Autodesk Fusion 360 part; units mm, degrees
(part 26 of 40)
  line L4946 (24.3039, -56.3229) -> (24.3478, -56.4711) construction
  line L4947 (24.3478, -56.4711) -> (24.3873, -56.6208) construction
  line L4948 (24.3873, -56.6208) -> (24.4241, -56.7714) construction
  line L4949 (24.4241, -56.7714) -> (24.4595, -56.9226) construction
  line L4950 (24.4595, -56.9226) -> (24.494, -57.0741) construction
  line L4951 (24.494, -57.0741) -> (24.5274, -57.226) construction
  line L4952 (24.5274, -57.226) -> (24.5594, -57.3783) construction
  line L4953 (24.5594, -57.3783) -> (24.5896, -57.5312) construction
  line L4954 (24.5896, -57.5312) -> (24.6176, -57.6848) construction
  line L4955 (24.6176, -57.6848) -> (24.6435, -57.8391) construction
  line L4956 (24.6435, -57.8391) -> (24.6674, -57.994) construction
  line L4957 (24.6674, -57.994) -> (24.6897, -58.1494) construction
  line L4958 (24.6897, -58.1494) -> (24.7105, -58.3052) construction
  line L4959 (24.7105, -58.3052) -> (24.7301, -58.4614) construction
  line L4960 (24.7301, -58.4614) -> (24.7485, -58.6179) construction
  line L4961 (24.7485, -58.6179) -> (24.7658, -58.7747) construction
  line L4962 (24.7658, -58.7747) -> (24.7818, -58.9318) construction
  line L4963 (24.7818, -58.9318) -> (24.7965, -59.0893) construction
  line L4964 (24.7965, -59.0893) -> (24.8098, -59.2471) construction
  line L4965 (24.8098, -59.2471) -> (24.8218, -59.4053) construction
  line L4966 (24.8218, -59.4053) -> (24.8325, -59.5638) construction
  line L4967 (24.8325, -59.5638) -> (24.842, -59.7226) construction
  line L4968 (24.842, -59.7226) -> (24.8504, -59.8817) construction
  line L4969 (24.8504, -59.8817) -> (24.8577, -60.0411) construction
  line L4970 (24.8577, -60.0411) -> (24.8638, -60.2007) construction
  line L4971 (24.8638, -60.2007) -> (24.8689, -60.3605) construction
  line L4972 (24.8689, -60.3605) -> (24.8729, -60.5206) construction
  line L4973 (24.8729, -60.5206) -> (24.8757, -60.6809) construction
  line L4974 (24.8757, -60.6809) -> (24.8776, -60.8415) construction
  line L4975 (24.8776, -60.8415) -> (24.8783, -61.0023) construction
  line L4976 (24.8783, -61.0023) -> (24.878, -61.1633) construction
  line L4977 (24.878, -61.1633) -> (24.8766, -61.3245) construction
  line L4978 (24.8766, -61.3245) -> (24.8742, -61.4859) construction
  line L4979 (24.8742, -61.4859) -> (24.8708, -61.6475) construction
  line L4980 (24.8708, -61.6475) -> (24.8665, -61.8093) construction
  line L4981 (24.8665, -61.8093) -> (24.8611, -61.9712) construction
  line L4982 (24.8611, -61.9712) -> (24.8548, -62.1334) construction
  line L4983 (24.8548, -62.1334) -> (24.8475, -62.2957) construction
  line L4984 (24.8475, -62.2957) -> (24.8392, -62.4581) construction
  line L4985 (24.8392, -62.4581) -> (24.83, -62.6207) construction
  line L4986 (24.83, -62.6207) -> (24.8199, -62.7835) construction
  line L4987 (24.8199, -62.7835) -> (24.8088, -62.9464) construction
  line L4988 (24.8088, -62.9464) -> (24.7967, -63.1095) construction
  line L4989 (24.7967, -63.1095) -> (24.7838, -63.2727) construction
  line L4990 (24.7838, -63.2727) -> (24.77, -63.436) construction
  line L4991 (24.77, -63.436) -> (24.7552, -63.5995) construction
  line L4992 (24.7552, -63.5995) -> (24.7396, -63.7631) construction
  line L4993 (24.7396, -63.7631) -> (24.723, -63.9268) construction
  line L4994 (24.723, -63.9268) -> (24.7056, -64.0906) construction
  line L4995 (24.7056, -64.0906) -> (24.6873, -64.2545) construction
  line L4996 (24.6873, -64.2545) -> (24.6681, -64.4185) construction
  line L4997 (24.6681, -64.4185) -> (24.648, -64.5826) construction
  line L4998 (24.648, -64.5826) -> (24.6271, -64.7468) construction
  line L4999 (24.6271, -64.7468) -> (24.6054, -64.9111) construction
  line L5000 (24.6054, -64.9111) -> (24.5828, -65.0755) construction
  line L5001 (24.5828, -65.0755) -> (24.5593, -65.24) construction
  line L5002 (24.5593, -65.24) -> (24.535, -65.4046) construction
  line L5003 (24.535, -65.4046) -> (24.5098, -65.5692) construction
  line L5004 (24.5098, -65.5692) -> (24.4839, -65.734) construction
  line L5005 (24.4839, -65.734) -> (24.4571, -65.8987) construction
  line L5006 (24.4571, -65.8987) -> (24.4294, -66.0636) construction
  line L5007 (24.4294, -66.0636) -> (24.401, -66.2285) construction
  line L5008 (24.401, -66.2285) -> (24.3718, -66.3935) construction
  line L5009 (24.3718, -66.3935) -> (24.3417, -66.5585) construction
  line L5010 (24.3417, -66.5585) -> (24.3108, -66.7236) construction
  line L5011 (24.3108, -66.7236) -> (24.2792, -66.8887) construction
  line L5012 (24.2792, -66.8887) -> (24.2532, -67.0208) construction
  line L5013 (24.2532, -67.0208) -> (24.2334, -67.1199) construction
  line L5014 (24.2334, -67.1199) -> (24.22, -67.186) construction
  line L5015 (24.22, -67.186) -> (24.2132, -67.2191) construction
  line L5016 (-59.1442, 5.5428) -> (-60.7685, 5.6951)
  line L5017 (-30.2798, 51.1066) -> (-31.1115, 52.5103)
  line L5018 (57.9623, -13.005) -> (59.5542, -13.3622)
  line L5019 (-13.005, 57.9623) -> (-13.3622, 59.5542)
  arc A123 (-54.5366, 23.5481) -> (-51.9354, 24.5301) centre (-53.7438, 25.3842) ccw
  arc A124 (56.9737, 7.2806) -> (59.1442, 5.5428) centre (58.9575, 7.5341) ccw
  arc A125 (-39.3784, 41.8132) -> (-39.2483, 44.5906) centre (-40.7496, 43.2692) ccw
  spline S67 degree 5 poles (-40.3263, 45.8153) (-40.3467, 45.8385) (-40.3868, 45.8854) (-40.4451, 45.9573) (-40.5192, 46.056) (-40.6066, 46.1833) (-40.6904, 46.3135) (-40.772, 46.4454) (-40.8524, 46.5782) (-40.932, 46.7117) (-41.0107, 46.8458) (-41.0883, 46.9807) (-41.1642, 47.1168) (-41.2383, 47.2543) (-41.3106, 47.393) (-41.3813, 47.5329) (-41.4504, 47.6738) (-41.5184, 47.8156) (-41.5853, 47.9581) (-41.6512, 48.1012) (-41.716, 48.245) (-41.7798, 48.3895) (-41.8424, 48.5347) (-41.9039, 48.6807) (-41.9642, 48.8274) (-42.0234, 48.9749) (-42.0815, 49.123) (-42.1386, 49.2717) (-42.1947, 49.421) (-42.2499, 49.5709) (-42.3041, 49.7214) (-42.3574, 49.8724) (-42.4097, 50.024) (-42.461, 50.1761) (-42.5114, 50.3288) (-42.5608, 50.482) (-42.6094, 50.6358) (-42.657, 50.79) (-42.7037, 50.9447) (-42.7495, 51.0999) (-42.7945, 51.2556) (-42.8386, 51.4118) (-42.8818, 51.5684) (-42.9241, 51.7255) (-42.9656, 51.883) (-43.0063, 52.0409) (-43.0461, 52.1993) (-43.085, 52.3581) (-43.1231, 52.5173) (-43.1604, 52.6769) (-43.1969, 52.8369) (-43.2326, 52.9973) (-43.2674, 53.1581) (-43.3015, 53.3193) (-43.3347, 53.4809) (-43.3672, 53.6428) (-43.3988, 53.8051) (-43.4297, 53.9677) (-43.4597, 54.1307) (-43.489, 54.294) (-43.5175, 54.4577) (-43.5453, 54.6217) (-43.5723, 54.7861) (-43.5984, 54.9508) (-43.6239, 55.1158) (-43.6486, 55.2811) (-43.6725, 55.4467) (-43.6956, 55.6126) (-43.718, 55.7789) (-43.7397, 55.9454) (-43.7606, 56.1122) (-43.7767, 56.2459) (-43.7885, 56.3463) (-43.7962, 56.4133) (-43.8, 56.4469) knots 0 0 0 0 0 0 0.01428571 0.02857143 0.04285714 0.05714286 0.07142857 0.08571429 0.1 0.11428571 0.12857143 0.14285714 0.15714286 0.17142857 0.18571429 0.2 0.21428571 0.22857143 0.24285714 0.25714286 0.27142857 0.28571429 0.3 0.31428571 0.32857143 0.34285714 0.35714286 0.37142857 0.38571429 0.4 0.41428571 0.42857143 0.44285714 0.45714286 0.47142857 0.48571429 0.5 0.51428571 0.52857143 0.54285714 0.55714286 0.57142857 0.58571429 0.6 0.61428571 0.62857143 0.64285714 0.65714286 0.67142857 0.68571429 0.7 0.71428571 0.72857143 0.74285714 0.75714286 0.77142857 0.78571429 0.8 0.81428571 0.82857143 0.84285714 0.85714286 0.87142857 0.88571429 0.9 0.91428571 0.92857143 0.94285714 0.95714286 0.97142857 0.98571429 1 1 1 1 1 1
  line L5020 (-40.3263, 45.8153) -> (-40.3467, 45.8385) construction
  line L5021 (-40.3467, 45.8385) -> (-40.3868, 45.8854) construction
  line L5022 (-40.3868, 45.8854) -> (-40.4451, 45.9573) construction
  line L5023 (-40.4451, 45.9573) -> (-40.5192, 46.056) construction
  line L5024 (-40.5192, 46.056) -> (-40.6066, 46.1833) construction
  line L5025 (-40.6066, 46.1833) -> (-40.6904, 46.3135) construction
  line L5026 (-40.6904, 46.3135) -> (-40.772, 46.4454) construction
  line L5027 (-40.772, 46.4454) -> (-40.8524, 46.5782) construction
  line L5028 (-40.8524, 46.5782) -> (-40.932, 46.7117) construction
  line L5029 (-40.932, 46.7117) -> (-41.0107, 46.8458) construction
  line L5030 (-41.0107, 46.8458) -> (-41.0883, 46.9807) construction
  line L5031 (-41.0883, 46.9807) -> (-41.1642, 47.1168) construction
  line L5032 (-41.1642, 47.1168) -> (-41.2383, 47.2543) construction
  line L5033 (-41.2383, 47.2543) -> (-41.3106, 47.393) construction
  line L5034 (-41.3106, 47.393) -> (-41.3813, 47.5329) construction
  line L5035 (-41.3813, 47.5329) -> (-41.4504, 47.6738) construction
  line L5036 (-41.4504, 47.6738) -> (-41.5184, 47.8156) construction
  line L5037 (-41.5184, 47.8156) -> (-41.5853, 47.9581) construction
  line L5038 (-41.5853, 47.9581) -> (-41.6512, 48.1012) construction
  line L5039 (-41.6512, 48.1012) -> (-41.716, 48.245) construction
  line L5040 (-41.716, 48.245) -> (-41.7798, 48.3895) construction
  line L5041 (-41.7798, 48.3895) -> (-41.8424, 48.5347) construction
  line L5042 (-41.8424, 48.5347) -> (-41.9039, 48.6807) construction
  line L5043 (-41.9039, 48.6807) -> (-41.9642, 48.8274) construction
  line L5044 (-41.9642, 48.8274) -> (-42.0234, 48.9749) construction
  line L5045 (-42.0234, 48.9749) -> (-42.0815, 49.123) construction
  line L5046 (-42.0815, 49.123) -> (-42.1386, 49.2717) construction
  line L5047 (-42.1386, 49.2717) -> (-42.1947, 49.421) construction
  line L5048 (-42.1947, 49.421) -> (-42.2499, 49.5709) construction
  line L5049 (-42.2499, 49.5709) -> (-42.3041, 49.7214) construction
  line L5050 (-42.3041, 49.7214) -> (-42.3574, 49.8724) construction
  line L5051 (-42.3574, 49.8724) -> (-42.4097, 50.024) construction
  line L5052 (-42.4097, 50.024) -> (-42.461, 50.1761) construction
  line L5053 (-42.461, 50.1761) -> (-42.5114, 50.3288) construction
  line L5054 (-42.5114, 50.3288) -> (-42.5608, 50.482) construction
  line L5055 (-42.5608, 50.482) -> (-42.6094, 50.6358) construction
  line L5056 (-42.6094, 50.6358) -> (-42.657, 50.79) construction
  line L5057 (-42.657, 50.79) -> (-42.7037, 50.9447) construction
  line L5058 (-42.7037, 50.9447) -> (-42.7495, 51.0999) construction
  line L5059 (-42.7495, 51.0999) -> (-42.7945, 51.2556) construction
  line L5060 (-42.7945, 51.2556) -> (-42.8386, 51.4118) construction
  line L5061 (-42.8386, 51.4118) -> (-42.8818, 51.5684) construction
  line L5062 (-42.8818, 51.5684) -> (-42.9241, 51.7255) construction
  line L5063 (-42.9241, 51.7255) -> (-42.9656, 51.883) construction
  line L5064 (-42.9656, 51.883) -> (-43.0063, 52.0409) construction
  line L5065 (-43.0063, 52.0409) -> (-43.0461, 52.1993) construction
  line L5066 (-43.0461, 52.1993) -> (-43.085, 52.3581) construction
  line L5067 (-43.085, 52.3581) -> (-43.1231, 52.5173) construction
  line L5068 (-43.1231, 52.5173) -> (-43.1604, 52.6769) construction
  line L5069 (-43.1604, 52.6769) -> (-43.1969, 52.8369) construction
  line L5070 (-43.1969, 52.8369) -> (-43.2326, 52.9973) construction
  line L5071 (-43.2326, 52.9973) -> (-43.2674, 53.1581) construction
  line L5072 (-43.2674, 53.1581) -> (-43.3015, 53.3193) construction
  line L5073 (-43.3015, 53.3193) -> (-43.3347, 53.4809) construction
  line L5074 (-43.3347, 53.4809) -> (-43.3672, 53.6428) construction
  line L5075 (-43.3672, 53.6428) -> (-43.3988, 53.8051) construction
  line L5076 (-43.3988, 53.8051) -> (-43.4297, 53.9677) construction
  line L5077 (-43.4297, 53.9677) -> (-43.4597, 54.1307) construction
  line L5078 (-43.4597, 54.1307) -> (-43.489, 54.294) construction
  line L5079 (-43.489, 54.294) -> (-43.5175, 54.4577) construction
  line L5080 (-43.5175, 54.4577) -> (-43.5453, 54.6217) construction
  line L5081 (-43.5453, 54.6217) -> (-43.5723, 54.7861) construction
  line L5082 (-43.5723, 54.7861) -> (-43.5984, 54.9508) construction
  line L5083 (-43.5984, 54.9508) -> (-43.6239, 55.1158) construction
  line L5084 (-43.6239, 55.1158) -> (-43.6486, 55.2811) construction
  line L5085 (-43.6486, 55.2811) -> (-43.6725, 55.4467) construction
  line L5086 (-43.6725, 55.4467) -> (-43.6956, 55.6126) construction
  line L5087 (-43.6956, 55.6126) -> (-43.718, 55.7789) construction
  line L5088 (-43.718, 55.7789) -> (-43.7397, 55.9454) construction
  line L5089 (-43.7397, 55.9454) -> (-43.7606, 56.1122) construction
  line L5090 (-43.7606, 56.1122) -> (-43.7767, 56.2459) construction
  line L5091 (-43.7767, 56.2459) -> (-43.7885, 56.3463) construction
  line L5092 (-43.7885, 56.3463) -> (-43.7962, 56.4133) construction
  line L5093 (-43.7962, 56.4133) -> (-43.8, 56.4469) construction
  arc A126 (24.2132, 67.2191) -> (19.9215, 68.6136) centre (0, 0) ccw
  spline S68 degree 5 poles (5.6951, 60.7685) (5.6979, 60.7993) (5.7029, 60.8609) (5.7078, 60.9533) (5.7097, 61.0766) (5.7056, 61.231) (5.6969, 61.3856) (5.6854, 61.5403) (5.6723, 61.695) (5.6583, 61.8498) (5.6431, 62.0045) (5.6265, 62.1593) (5.608, 62.314) (5.5871, 62.4688) (5.5641, 62.6235) (5.539, 62.7782) (5.5121, 62.9329) (5.4838, 63.0875) (5.4542, 63.2421) (5.4233, 63.3966) (5.3913, 63.5511) (5.3579, 63.7055) (5.3232, 63.8598) (5.2871, 64.014) (5.2497, 64.1682) (5.2109, 64.3222) (5.1709, 64.4762) (5.1297, 64.6301) (5.0873, 64.7839) (5.0439, 64.9376) (4.9993, 65.0912) (4.9536, 65.2447) (4.9068, 65.398) (4.8589, 65.5513) (4.8099, 65.7044) (4.7599, 65.8574) (4.7087, 66.0103) (4.6566, 66.1631) (4.6035, 66.3158) (4.5493, 66.4683) (4.4942, 66.6206) (4.438, 66.7729) (4.381, 66.925) (4.3229, 67.077) (4.2639, 67.2288) (4.2039, 67.3804) (4.143, 67.532) (4.0812, 67.6833) (4.0185, 67.8345) (3.9548, 67.9856) (3.8903, 68.1365) (3.8249, 68.2872) (3.7585, 68.4378) (3.6913, 68.5882) (3.6233, 68.7384) (3.5543, 68.8885) (3.4846, 69.0384) (3.4139, 69.1881) (3.3425, 69.3376) (3.2701, 69.487) (3.197, 69.6362) (3.123, 69.7852) (3.0482, 69.934) (2.9726, 70.0826) (2.8962, 70.2311) (2.819, 70.3793) (2.741, 70.5274) (2.6622, 70.6752) (2.5826, 70.8229) (2.5023, 70.9703) (2.4211, 71.1176) (2.3556, 71.2352) (2.3061, 71.3234) (2.2729, 71.3821) (2.2563, 71.4115) knots 0 0 0 0 0 0 0.01428571 0.02857143 0.04285714 0.05714286 0.07142857 0.08571429 0.1 0.11428571 0.12857143 0.14285714 0.15714286 0.17142857 0.18571429 0.2 0.21428571 0.22857143 0.24285714 0.25714286 0.27142857 0.28571429 0.3 0.31428571 0.32857143 0.34285714 0.35714286 0.37142857 0.38571429 0.4 0.41428571 0.42857143 0.44285714 0.45714286 0.47142857 0.48571429 0.5 0.51428571 0.52857143 0.54285714 0.55714286 0.57142857 0.58571429 0.6 0.61428571 0.62857143 0.64285714 0.65714286 0.67142857 0.68571429 0.7 0.71428571 0.72857143 0.74285714 0.75714286 0.77142857 0.78571429 0.8 0.81428571 0.82857143 0.84285714 0.85714286 0.87142857 0.88571429 0.9 0.91428571 0.92857143 0.94285714 0.95714286 0.97142857 0.98571429 1 1 1 1 1 1
  line L5094 (5.6951, 60.7685) -> (5.6979, 60.7993) construction
  line L5095 (5.6979, 60.7993) -> (5.7029, 60.8609) construction
  line L5096 (5.7029, 60.8609) -> (5.7078, 60.9533) construction
  line L5097 (5.7078, 60.9533) -> (5.7097, 61.0766) construction
  line L5098 (5.7097, 61.0766) -> (5.7056, 61.231) construction
  line L5099 (5.7056, 61.231) -> (5.6969, 61.3856) construction
  line L5100 (5.6969, 61.3856) -> (5.6854, 61.5403) construction
  line L5101 (5.6854, 61.5403) -> (5.6723, 61.695) construction
  line L5102 (5.6723, 61.695) -> (5.6583, 61.8498) construction
  line L5103 (5.6583, 61.8498) -> (5.6431, 62.0045) construction
  line L5104 (5.6431, 62.0045) -> (5.6265, 62.1593) construction
  line L5105 (5.6265, 62.1593) -> (5.608, 62.314) construction
  line L5106 (5.608, 62.314) -> (5.5871, 62.4688) construction
  line L5107 (5.5871, 62.4688) -> (5.5641, 62.6235) construction
  line L5108 (5.5641, 62.6235) -> (5.539, 62.7782) construction
  line L5109 (5.539, 62.7782) -> (5.5121, 62.9329) construction
  line L5110 (5.5121, 62.9329) -> (5.4838, 63.0875) construction
  line L5111 (5.4838, 63.0875) -> (5.4542, 63.2421) construction
  line L5112 (5.4542, 63.2421) -> (5.4233, 63.3966) construction
  line L5113 (5.4233, 63.3966) -> (5.3913, 63.5511) construction
  line L5114 (5.3913, 63.5511) -> (5.3579, 63.7055) construction
  line L5115 (5.3579, 63.7055) -> (5.3232, 63.8598) construction
  line L5116 (5.3232, 63.8598) -> (5.2871, 64.014) construction
  line L5117 (5.2871, 64.014) -> (5.2497, 64.1682) construction
  line L5118 (5.2497, 64.1682) -> (5.2109, 64.3222) construction
  line L5119 (5.2109, 64.3222) -> (5.1709, 64.4762) construction
  line L5120 (5.1709, 64.4762) -> (5.1297, 64.6301) construction
  line L5121 (5.1297, 64.6301) -> (5.0873, 64.7839) construction
  line L5122 (5.0873, 64.7839) -> (5.0439, 64.9376) construction
  line L5123 (5.0439, 64.9376) -> (4.9993, 65.0912) construction
  line L5124 (4.9993, 65.0912) -> (4.9536, 65.2447) construction
  line L5125 (4.9536, 65.2447) -> (4.9068, 65.398) construction
  line L5126 (4.9068, 65.398) -> (4.8589, 65.5513) construction
  line L5127 (4.8589, 65.5513) -> (4.8099, 65.7044) construction
  line L5128 (4.8099, 65.7044) -> (4.7599, 65.8574) construction
  line L5129 (4.7599, 65.8574) -> (4.7087, 66.0103) construction
  line L5130 (4.7087, 66.0103) -> (4.6566, 66.1631) construction
  line L5131 (4.6566, 66.1631) -> (4.6035, 66.3158) construction
  line L5132 (4.6035, 66.3158) -> (4.5493, 66.4683) construction
  line L5133 (4.5493, 66.4683) -> (4.4942, 66.6206) construction
  line L5134 (4.4942, 66.6206) -> (4.438, 66.7729) construction
  line L5135 (4.438, 66.7729) -> (4.381, 66.925) construction
  line L5136 (4.381, 66.925) -> (4.3229, 67.077) construction
  line L5137 (4.3229, 67.077) -> (4.2639, 67.2288) construction
  line L5138 (4.2639, 67.2288) -> (4.2039, 67.3804) construction
  line L5139 (4.2039, 67.3804) -> (4.143, 67.532) construction
  line L5140 (4.143, 67.532) -> (4.0812, 67.6833) construction
  line L5141 (4.0812, 67.6833) -> (4.0185, 67.8345) construction
  line L5142 (4.0185, 67.8345) -> (3.9548, 67.9856) construction
  line L5143 (3.9548, 67.9856) -> (3.8903, 68.1365) construction
  line L5144 (3.8903, 68.1365) -> (3.8249, 68.2872) construction
  line L5145 (3.8249, 68.2872) -> (3.7585, 68.4378) construction
  line L5146 (3.7585, 68.4378) -> (3.6913, 68.5882) construction
  line L5147 (3.6913, 68.5882) -> (3.6233, 68.7384) construction
  line L5148 (3.6233, 68.7384) -> (3.5543, 68.8885) construction
  line L5149 (3.5543, 68.8885) -> (3.4846, 69.0384) construction
  line L5150 (3.4846, 69.0384) -> (3.4139, 69.1881) construction
  line L5151 (3.4139, 69.1881) -> (3.3425, 69.3376) construction
  line L5152 (3.3425, 69.3376) -> (3.2701, 69.487) construction
  line L5153 (3.2701, 69.487) -> (3.197, 69.6362) construction
  line L5154 (3.197, 69.6362) -> (3.123, 69.7852) construction
  line L5155 (3.123, 69.7852) -> (3.0482, 69.934) construction
  line L5156 (3.0482, 69.934) -> (2.9726, 70.0826) construction
  line L5157 (2.9726, 70.0826) -> (2.8962, 70.2311) construction
  line L5158 (2.8962, 70.2311) -> (2.819, 70.3793) construction
  line L5159 (2.819, 70.3793) -> (2.741, 70.5274) construction
  line L5160 (2.741, 70.5274) -> (2.6622, 70.6752) construction
  line L5161 (2.6622, 70.6752) -> (2.5826, 70.8229) construction
  line L5162 (2.5826, 70.8229) -> (2.5023, 70.9703) construction
  line L5163 (2.5023, 70.9703) -> (2.4211, 71.1176) construction
  line L5164 (2.4211, 71.1176) -> (2.3556, 71.2352) construction
  line L5165 (2.3556, 71.2352) -> (2.3061, 71.3234) construction
  line L5166 (2.3061, 71.3234) -> (2.2729, 71.3821) construction
  line L5167 (2.2729, 71.3821) -> (2.2563, 71.4115) construction
  arc A127 (-41.8132, -39.3784) -> (-44.5906, -39.2483) centre (-43.2692, -40.7496) ccw
  arc A128 (39.3784, -41.8132) -> (39.2483, -44.5906) centre (40.7496, -43.2692) ccw
  arc A129 (54.5366, -23.5481) -> (51.9354, -24.5301) centre (53.7438, -25.3842) ccw
  spline S69 degree 5 poles (-31.1115, 52.5103) (-31.1272, 52.5368) (-31.1594, 52.5895) (-31.2097, 52.6672) (-31.2807, 52.7681) (-31.3748, 52.8906) (-31.4727, 53.0106) (-31.5729, 53.1289) (-31.6744, 53.2464) (-31.7767, 53.3634) (-31.88, 53.4797) (-31.9844, 53.5951) (-32.0903, 53.7094) (-32.1981, 53.8224) (-32.3077, 53.934) (-32.419, 54.0444) (-32.5316, 54.1537) (-32.6455, 54.2622) (-32.7603, 54.3698) (-32.876, 54.4767) (-32.9927, 54.5828) (-33.1105, 54.6881) (-33.2292, 54.7926) (-33.3491, 54.8961) (-33.47, 54.9988) (-33.5919, 55.1007) (-33.7148, 55.2017) (-33.8386, 55.302) (-33.9633, 55.4015) (-34.0888, 55.5003) (-34.2151, 55.5984) (-34.3423, 55.6957) (-34.4703, 55.7923) (-34.5991, 55.8881) (-34.7288, 55.9832) (-34.8592, 56.0776) (-34.9905, 56.1712) (-35.1224, 56.2642) (-35.2552, 56.3564) (-35.3886, 56.448) (-35.5228, 56.5388) (-35.6577, 56.629) (-35.7933, 56.7185) (-35.9295, 56.8073) (-36.0665, 56.8955) (-36.2042, 56.9829) (-36.3425, 57.0697) (-36.4815, 57.1558) (-36.6211, 57.2413) (-36.7614, 57.3261) (-36.9023, 57.4102) (-37.0438, 57.4937) (-37.186, 57.5765) (-37.3288, 57.6587) (-37.4721, 57.7403) (-37.6161, 57.8212) (-37.7607, 57.9014) (-37.9058, 57.981) (-38.0515, 58.06) (-38.1978, 58.1383) (-38.3447, 58.216) (-38.4921, 58.2931) (-38.6401, 58.3695) (-38.7886, 58.4453) (-38.9377, 58.5205) (-39.0873, 58.595) (-39.2374, 58.669) (-39.3881, 58.7423) (-39.5393, 58.8149) (-39.6909, 58.887) (-39.8431, 58.9584) (-39.9653, 59.0151) (-40.0572, 59.0573) (-40.1185, 59.0853) (-40.1492, 59.0993) knots 0 0 0 0 0 0 0.01428571 0.02857143 0.04285714 0.05714286 0.07142857 0.08571429 0.1 0.11428571 0.12857143 0.14285714 0.15714286 0.17142857 0.18571429 0.2 0.21428571 0.22857143 0.24285714 0.25714286 0.27142857 0.28571429 0.3 0.31428571 0.32857143 0.34285714 0.35714286 0.37142857 0.38571429 0.4 0.41428571 0.42857143 0.44285714 0.45714286 0.47142857 0.48571429 0.5 0.51428571 0.52857143 0.54285714 0.55714286 0.57142857 0.58571429 0.6 0.61428571 0.62857143 0.64285714 0.65714286 0.67142857 0.68571429 0.7 0.71428571 0.72857143 0.74285714 0.75714286 0.77142857 0.78571429 0.8 0.81428571 0.82857143 0.84285714 0.85714286 0.87142857 0.88571429 0.9 0.91428571 0.92857143 0.94285714 0.95714286 0.97142857 0.98571429 1 1 1 1 1 1
  line L5168 (-31.1115, 52.5103) -> (-31.1272, 52.5368) construction
  line L5169 (-31.1272, 52.5368) -> (-31.1594, 52.5895) construction
  line L5170 (-31.1594, 52.5895) -> (-31.2097, 52.6672) construction
  line L5171 (-31.2097, 52.6672) -> (-31.2807, 52.7681) construction
  line L5172 (-31.2807, 52.7681) -> (-31.3748, 52.8906) construction
  line L5173 (-31.3748, 52.8906) -> (-31.4727, 53.0106) construction
  line L5174 (-31.4727, 53.0106) -> (-31.5729, 53.1289) construction
  line L5175 (-31.5729, 53.1289) -> (-31.6744, 53.2464) construction
  line L5176 (-31.6744, 53.2464) -> (-31.7767, 53.3634) construction
  line L5177 (-31.7767, 53.3634) -> (-31.88, 53.4797) construction
  line L5178 (-31.88, 53.4797) -> (-31.9844, 53.5951) construction
  line L5179 (-31.9844, 53.5951) -> (-32.0903, 53.7094) construction
  line L5180 (-32.0903, 53.7094) -> (-32.1981, 53.8224) construction
  line L5181 (-32.1981, 53.8224) -> (-32.3077, 53.934) construction
  line L5182 (-32.3077, 53.934) -> (-32.419, 54.0444) construction
  line L5183 (-32.419, 54.0444) -> (-32.5316, 54.1537) construction
  line L5184 (-32.5316, 54.1537) -> (-32.6455, 54.2622) construction
  line L5185 (-32.6455, 54.2622) -> (-32.7603, 54.3698) construction
  line L5186 (-32.7603, 54.3698) -> (-32.876, 54.4767) construction
  line L5187 (-32.876, 54.4767) -> (-32.9927, 54.5828) construction
  line L5188 (-32.9927, 54.5828) -> (-33.1105, 54.6881) construction
  line L5189 (-33.1105, 54.6881) -> (-33.2292, 54.7926) construction
  line L5190 (-33.2292, 54.7926) -> (-33.3491, 54.8961) construction
  line L5191 (-33.3491, 54.8961) -> (-33.47, 54.9988) construction
  line L5192 (-33.47, 54.9988) -> (-33.5919, 55.1007) construction
  line L5193 (-33.5919, 55.1007) -> (-33.7148, 55.2017) construction
  line L5194 (-33.7148, 55.2017) -> (-33.8386, 55.302) construction
  line L5195 (-33.8386, 55.302) -> (-33.9633, 55.4015) construction
  line L5196 (-33.9633, 55.4015) -> (-34.0888, 55.5003) construction
  line L5197 (-34.0888, 55.5003) -> (-34.2151, 55.5984) construction
  line L5198 (-34.2151, 55.5984) -> (-34.3423, 55.6957) construction
  line L5199 (-34.3423, 55.6957) -> (-34.4703, 55.7923) construction
  line L5200 (-34.4703, 55.7923) -> (-34.5991, 55.8881) construction
  line L5201 (-34.5991, 55.8881) -> (-34.7288, 55.9832) construction
  line L5202 (-34.7288, 55.9832) -> (-34.8592, 56.0776) construction
  line L5203 (-34.8592, 56.0776) -> (-34.9905, 56.1712) construction
  line L5204 (-34.9905, 56.1712) -> (-35.1224, 56.2642) construction
  line L5205 (-35.1224, 56.2642) -> (-35.2552, 56.3564) construction
  line L5206 (-35.2552, 56.3564) -> (-35.3886, 56.448) construction
  line L5207 (-35.3886, 56.448) -> (-35.5228, 56.5388) construction
  line L5208 (-35.5228, 56.5388) -> (-35.6577, 56.629) construction
  line L5209 (-35.6577, 56.629) -> (-35.7933, 56.7185) construction
  line L5210 (-35.7933, 56.7185) -> (-35.9295, 56.8073) construction
  line L5211 (-35.9295, 56.8073) -> (-36.0665, 56.8955) construction
  line L5212 (-36.0665, 56.8955) -> (-36.2042, 56.9829) construction
  line L5213 (-36.2042, 56.9829) -> (-36.3425, 57.0697) construction
  line L5214 (-36.3425, 57.0697) -> (-36.4815, 57.1558) construction
  line L5215 (-36.4815, 57.1558) -> (-36.6211, 57.2413) construction
  line L5216 (-36.6211, 57.2413) -> (-36.7614, 57.3261) construction
  line L5217 (-36.7614, 57.3261) -> (-36.9023, 57.4102) construction
  line L5218 (-36.9023, 57.4102) -> (-37.0438, 57.4937) construction
  line L5219 (-37.0438, 57.4937) -> (-37.186, 57.5765) construction
  line L5220 (-37.186, 57.5765) -> (-37.3288, 57.6587) construction
  line L5221 (-37.3288, 57.6587) -> (-37.4721, 57.7403) construction
  line L5222 (-37.4721, 57.7403) -> (-37.6161, 57.8212) construction
  line L5223 (-37.6161, 57.8212) -> (-37.7607, 57.9014) construction
  line L5224 (-37.7607, 57.9014) -> (-37.9058, 57.981) construction
  line L5225 (-37.9058, 57.981) -> (-38.0515, 58.06) construction
  line L5226 (-38.0515, 58.06) -> (-38.1978, 58.1383) construction
  line L5227 (-38.1978, 58.1383) -> (-38.3447, 58.216) construction
  line L5228 (-38.3447, 58.216) -> (-38.4921, 58.2931) construction
  line L5229 (-38.4921, 58.2931) -> (-38.6401, 58.3695) construction
  line L5230 (-38.6401, 58.3695) -> (-38.7886, 58.4453) construction
  line L5231 (-38.7886, 58.4453) -> (-38.9377, 58.5205) construction
  line L5232 (-38.9377, 58.5205) -> (-39.0873, 58.595) construction
  line L5233 (-39.0873, 58.595) -> (-39.2374, 58.669) construction
  line L5234 (-39.2374, 58.669) -> (-39.3881, 58.7423) construction
  line L5235 (-39.3881, 58.7423) -> (-39.5393, 58.8149) construction
  line L5236 (-39.5393, 58.8149) -> (-39.6909, 58.887) construction
  line L5237 (-39.6909, 58.887) -> (-39.8431, 58.9584) construction
  line L5238 (-39.8431, 58.9584) -> (-39.9653, 59.0151) construction
  line L5239 (-39.9653, 59.0151) -> (-40.0572, 59.0573) construction
  line L5240 (-40.0572, 59.0573) -> (-40.1185, 59.0853) construction
  line L5241 (-40.1185, 59.0853) -> (-40.1492, 59.0993) construction
  arc A130 (41.8132, 39.3784) -> (44.5906, 39.2483) centre (43.2692, 40.7496) ccw
  spline S70 degree 5 poles (5.6951, -60.7685) (5.6979, -60.7993) (5.7029, -60.8609) (5.7078, -60.9533) (5.7097, -61.0766) (5.7056, -61.231) (5.6969, -61.3856) (5.6854, -61.5403) (5.6723, -61.695) (5.6583, -61.8498) (5.6431, -62.0045) (5.6265, -62.1593) (5.608, -62.314) (5.5871, -62.4688) (5.5641, -62.6235) (5.539, -62.7782) (5.5121, -62.9329) (5.4838, -63.0875) (5.4542, -63.2421) (5.4233, -63.3966) (5.3913, -63.5511) (5.3579, -63.7055) (5.3232, -63.8598) (5.2871, -64.014) (5.2497, -64.1682) (5.2109, -64.3222) (5.1709, -64.4762) (5.1297, -64.6301) (5.0873, -64.7839) (5.0439, -64.9376) (4.9993, -65.0912) (4.9536, -65.2447) (4.9068, -65.398) (4.8589, -65.5513) (4.8099, -65.7044) (4.7599, -65.8574) (4.7087, -66.0103) (4.6566, -66.1631) (4.6035, -66.3158) (4.5493, -66.4683) (4.4942, -66.6206) (4.438, -66.7729) (4.381, -66.925) (4.3229, -67.077) (4.2639, -67.2288) (4.2039, -67.3804) (4.143, -67.532) (4.0812, -67.6833) (4.0185, -67.8345) (3.9548, -67.9856) (3.8903, -68.1365) (3.8249, -68.2872) (3.7585, -68.4378) (3.6913, -68.5882) (3.6233, -68.7384) (3.5543, -68.8885) (3.4846, -69.0384) (3.4139, -69.1881) (3.3425, -69.3376) (3.2701, -69.487) (3.197, -69.6362) (3.123, -69.7852) (3.0482, -69.934) (2.9726, -70.0826) (2.8962, -70.2311) (2.819, -70.3793) (2.741, -70.5274) (2.6622, -70.6752) (2.5826, -70.8229) (2.5023, -70.9703) (2.4211, -71.1176) (2.3556, -71.2352) (2.3061, -71.3234) (2.2729, -71.3821) (2.2563, -71.4115) knots 0 0 0 0 0 0 0.01428571 0.02857143 0.04285714 0.05714286 0.07142857 0.08571429 0.1 0.11428571 0.12857143 0.14285714 0.15714286 0.17142857 0.18571429 0.2 0.21428571 0.22857143 0.24285714 0.25714286 0.27142857 0.28571429 0.3 0.31428571 0.32857143 0.34285714 0.35714286 0.37142857 0.38571429 0.4 0.41428571 0.42857143 0.44285714 0.45714286 0.47142857 0.48571429 0.5 0.51428571 0.52857143 0.54285714 0.55714286 0.57142857 0.58571429 0.6 0.61428571 0.62857143 0.64285714 0.65714286 0.67142857 0.68571429 0.7 0.71428571 0.72857143 0.74285714 0.75714286 0.77142857 0.78571429 0.8 0.81428571 0.82857143 0.84285714 0.85714286 0.87142857 0.88571429 0.9 0.91428571 0.92857143 0.94285714 0.95714286 0.97142857 0.98571429 1 1 1 1 1 1
  line L5242 (5.6951, -60.7685) -> (5.6979, -60.7993) construction
  line L5243 (5.6979, -60.7993) -> (5.7029, -60.8609) construction
  line L5244 (5.7029, -60.8609) -> (5.7078, -60.9533) construction
  line L5245 (5.7078, -60.9533) -> (5.7097, -61.0766) construction
  line L5246 (5.7097, -61.0766) -> (5.7056, -61.231) construction
  line L5247 (5.7056, -61.231) -> (5.6969, -61.3856) construction
  line L5248 (5.6969, -61.3856) -> (5.6854, -61.5403) construction
  line L5249 (5.6854, -61.5403) -> (5.6723, -61.695) construction
  line L5250 (5.6723, -61.695) -> (5.6583, -61.8498) construction
  line L5251 (5.6583, -61.8498) -> (5.6431, -62.0045) construction
  line L5252 (5.6431, -62.0045) -> (5.6265, -62.1593) construction
  line L5253 (5.6265, -62.1593) -> (5.608, -62.314) construction
  line L5254 (5.608, -62.314) -> (5.5871, -62.4688) construction
  line L5255 (5.5871, -62.4688) -> (5.5641, -62.6235) construction
  line L5256 (5.5641, -62.6235) -> (5.539, -62.7782) construction
  line L5257 (5.539, -62.7782) -> (5.5121, -62.9329) construction
  line L5258 (5.5121, -62.9329) -> (5.4838, -63.0875) construction
  line L5259 (5.4838, -63.0875) -> (5.4542, -63.2421) construction
  line L5260 (5.4542, -63.2421) -> (5.4233, -63.3966) construction
  line L5261 (5.4233, -63.3966) -> (5.3913, -63.5511) construction
  line L5262 (5.3913, -63.5511) -> (5.3579, -63.7055) construction
  line L5263 (5.3579, -63.7055) -> (5.3232, -63.8598) construction
  line L5264 (5.3232, -63.8598) -> (5.2871, -64.014) construction
  line L5265 (5.2871, -64.014) -> (5.2497, -64.1682) construction
  line L5266 (5.2497, -64.1682) -> (5.2109, -64.3222) construction
  line L5267 (5.2109, -64.3222) -> (5.1709, -64.4762) construction
  line L5268 (5.1709, -64.4762) -> (5.1297, -64.6301) construction
  line L5269 (5.1297, -64.6301) -> (5.0873, -64.7839) construction
  line L5270 (5.0873, -64.7839) -> (5.0439, -64.9376) construction
  line L5271 (5.0439, -64.9376) -> (4.9993, -65.0912) construction
  line L5272 (4.9993, -65.0912) -> (4.9536, -65.2447) construction
  line L5273 (4.9536, -65.2447) -> (4.9068, -65.398) construction
  line L5274 (4.9068, -65.398) -> (4.8589, -65.5513) construction
  line L5275 (4.8589, -65.5513) -> (4.8099, -65.7044) construction
  line L5276 (4.8099, -65.7044) -> (4.7599, -65.8574) construction
  line L5277 (4.7599, -65.8574) -> (4.7087, -66.0103) construction
  line L5278 (4.7087, -66.0103) -> (4.6566, -66.1631) construction
  line L5279 (4.6566, -66.1631) -> (4.6035, -66.3158) construction
  line L5280 (4.6035, -66.3158) -> (4.5493, -66.4683) construction
  line L5281 (4.5493, -66.4683) -> (4.4942, -66.6206) construction
  line L5282 (4.4942, -66.6206) -> (4.438, -66.7729) construction
  line L5283 (4.438, -66.7729) -> (4.381, -66.925) construction
  line L5284 (4.381, -66.925) -> (4.3229, -67.077) construction
  line L5285 (4.3229, -67.077) -> (4.2639, -67.2288) construction
  line L5286 (4.2639, -67.2288) -> (4.2039, -67.3804) construction
  line L5287 (4.2039, -67.3804) -> (4.143, -67.532) construction
  line L5288 (4.143, -67.532) -> (4.0812, -67.6833) construction
  line L5289 (4.0812, -67.6833) -> (4.0185, -67.8345) construction
  line L5290 (4.0185, -67.8345) -> (3.9548, -67.9856) construction
  line L5291 (3.9548, -67.9856) -> (3.8903, -68.1365) construction
  line L5292 (3.8903, -68.1365) -> (3.8249, -68.2872) construction
  line L5293 (3.8249, -68.2872) -> (3.7585, -68.4378) construction
  line L5294 (3.7585, -68.4378) -> (3.6913, -68.5882) construction
  line L5295 (3.6913, -68.5882) -> (3.6233, -68.7384) construction
  line L5296 (3.6233, -68.7384) -> (3.5543, -68.8885) construction
  line L5297 (3.5543, -68.8885) -> (3.4846, -69.0384) construction
  line L5298 (3.4846, -69.0384) -> (3.4139, -69.1881) construction
  line L5299 (3.4139, -69.1881) -> (3.3425, -69.3376) construction
  line L5300 (3.3425, -69.3376) -> (3.2701, -69.487) construction
  line L5301 (3.2701, -69.487) -> (3.197, -69.6362) construction
  line L5302 (3.197, -69.6362) -> (3.123, -69.7852) construction
  line L5303 (3.123, -69.7852) -> (3.0482, -69.934) construction
  line L5304 (3.0482, -69.934) -> (2.9726, -70.0826) construction
  line L5305 (2.9726, -70.0826) -> (2.8962, -70.2311) construction
  line L5306 (2.8962, -70.2311) -> (2.819, -70.3793) construction
  line L5307 (2.819, -70.3793) -> (2.741, -70.5274) construction
  line L5308 (2.741, -70.5274) -> (2.6622, -70.6752) construction
  line L5309 (2.6622, -70.6752) -> (2.5826, -70.8229) construction
  line L5310 (2.5826, -70.8229) -> (2.5023, -70.9703) construction
  line L5311 (2.5023, -70.9703) -> (2.4211, -71.1176) construction
  line L5312 (2.4211, -71.1176) -> (2.3556, -71.2352) construction
  line L5313 (2.3556, -71.2352) -> (2.3061, -71.3234) construction
  line L5314 (2.3061, -71.3234) -> (2.2729, -71.3821) construction
  line L5315 (2.2729, -71.3821) -> (2.2563, -71.4115) construction
  arc A131 (2.2563, 71.4115) -> (-2.2563, 71.4115) centre (0, 0) ccw
  spline S71 degree 5 poles (52.5103, 31.1115) (52.5368, 31.1272) (52.5895, 31.1594) (52.6672, 31.2097) (52.7681, 31.2807) (52.8906, 31.3748) (53.0106, 31.4727) (53.1289, 31.5729) (53.2464, 31.6744) (53.3634, 31.7767) (53.4797, 31.88) (53.5951, 31.9844) (53.7094, 32.0903) (53.8224, 32.1981) (53.934, 32.3077) (54.0444, 32.419) (54.1537, 32.5316) (54.2622, 32.6455) (54.3698, 32.7603) (54.4767, 32.876) (54.5828, 32.9927) (54.6881, 33.1105) (54.7926, 33.2292) (54.8961, 33.3491) (54.9988, 33.47) (55.1007, 33.5919) (55.2017, 33.7148) (55.302, 33.8386) (55.4015, 33.9633) (55.5003, 34.0888) (55.5984, 34.2151) (55.6957, 34.3423) (55.7923, 34.4703) (55.8881, 34.5991) (55.9832, 34.7288) (56.0776, 34.8592) (56.1712, 34.9905) (56.2642, 35.1224) (56.3564, 35.2552) (56.448, 35.3886) (56.5388, 35.5228) (56.629, 35.6577) (56.7185, 35.7933) (56.8073, 35.9295) (56.8955, 36.0665) (56.9829, 36.2042) (57.0697, 36.3425) (57.1558, 36.4815) (57.2413, 36.6211) (57.3261, 36.7614) (57.4102, 36.9023) (57.4937, 37.0438) (57.5765, 37.186) (57.6587, 37.3288) (57.7403, 37.4721) (57.8212, 37.6161) (57.9014, 37.7607) (57.981, 37.9058) (58.06, 38.0515) (58.1383, 38.1978) (58.216, 38.3447) (58.2931, 38.4921) (58.3695, 38.6401) (58.4453, 38.7886) (58.5205, 38.9377) (58.595, 39.0873) (58.669, 39.2374) (58.7423, 39.3881) (58.8149, 39.5393) (58.887, 39.6909) (58.9584, 39.8431) (59.0151, 39.9653) (59.0573, 40.0572) (59.0853, 40.1185) (59.0993, 40.1492) knots 0 0 0 0 0 0 0.01428571 0.02857143 0.04285714 0.05714286 0.07142857 0.08571429 0.1 0.11428571 0.12857143 0.14285714 0.15714286 0.17142857 0.18571429 0.2 0.21428571 0.22857143 0.24285714 0.25714286 0.27142857 0.28571429 0.3 0.31428571 0.32857143 0.34285714 0.35714286 0.37142857 0.38571429 0.4 0.41428571 0.42857143 0.44285714 0.45714286 0.47142857 0.48571429 0.5 0.51428571 0.52857143 0.54285714 0.55714286 0.57142857 0.58571429 0.6 0.61428571 0.62857143 0.64285714 0.65714286 0.67142857 0.68571429 0.7 0.71428571 0.72857143 0.74285714 0.75714286 0.77142857 0.78571429 0.8 0.81428571 0.82857143 0.84285714 0.85714286 0.87142857 0.88571429 0.9 0.91428571 0.92857143 0.94285714 0.95714286 0.97142857 0.98571429 1 1 1 1 1 1
  line L5316 (52.5103, 31.1115) -> (52.5368, 31.1272) construction
  line L5317 (52.5368, 31.1272) -> (52.5895, 31.1594) construction
  line L5318 (52.5895, 31.1594) -> (52.6672, 31.2097) construction
  line L5319 (52.6672, 31.2097) -> (52.7681, 31.2807) construction
  line L5320 (52.7681, 31.2807) -> (52.8906, 31.3748) construction
  line L5321 (52.8906, 31.3748) -> (53.0106, 31.4727) construction
  line L5322 (53.0106, 31.4727) -> (53.1289, 31.5729) construction
  line L5323 (53.1289, 31.5729) -> (53.2464, 31.6744) construction
  line L5324 (53.2464, 31.6744) -> (53.3634, 31.7767) construction
  line L5325 (53.3634, 31.7767) -> (53.4797, 31.88) construction
  line L5326 (53.4797, 31.88) -> (53.5951, 31.9844) construction
  line L5327 (53.5951, 31.9844) -> (53.7094, 32.0903) construction
  line L5328 (53.7094, 32.0903) -> (53.8224, 32.1981) construction
  line L5329 (53.8224, 32.1981) -> (53.934, 32.3077) construction
  line L5330 (53.934, 32.3077) -> (54.0444, 32.419) construction
  line L5331 (54.0444, 32.419) -> (54.1537, 32.5316) construction
  line L5332 (54.1537, 32.5316) -> (54.2622, 32.6455) construction
  line L5333 (54.2622, 32.6455) -> (54.3698, 32.7603) construction
  line L5334 (54.3698, 32.7603) -> (54.4767, 32.876) construction
  line L5335 (54.4767, 32.876) -> (54.5828, 32.9927) construction
  line L5336 (54.5828, 32.9927) -> (54.6881, 33.1105) construction
  line L5337 (54.6881, 33.1105) -> (54.7926, 33.2292) construction
  line L5338 (54.7926, 33.2292) -> (54.8961, 33.3491) construction
  line L5339 (54.8961, 33.3491) -> (54.9988, 33.47) construction
  line L5340 (54.9988, 33.47) -> (55.1007, 33.5919) construction
  line L5341 (55.1007, 33.5919) -> (55.2017, 33.7148) construction
  line L5342 (55.2017, 33.7148) -> (55.302, 33.8386) construction
  line L5343 (55.302, 33.8386) -> (55.4015, 33.9633) construction
  line L5344 (55.4015, 33.9633) -> (55.5003, 34.0888) construction
  line L5345 (55.5003, 34.0888) -> (55.5984, 34.2151) construction
  line L5346 (55.5984, 34.2151) -> (55.6957, 34.3423) construction
  line L5347 (55.6957, 34.3423) -> (55.7923, 34.4703) construction
  line L5348 (55.7923, 34.4703) -> (55.8881, 34.5991) construction
  line L5349 (55.8881, 34.5991) -> (55.9832, 34.7288) construction
  line L5350 (55.9832, 34.7288) -> (56.0776, 34.8592) construction
  line L5351 (56.0776, 34.8592) -> (56.1712, 34.9905) construction
  line L5352 (56.1712, 34.9905) -> (56.2642, 35.1224) construction
  line L5353 (56.2642, 35.1224) -> (56.3564, 35.2552) construction
  line L5354 (56.3564, 35.2552) -> (56.448, 35.3886) construction
  line L5355 (56.448, 35.3886) -> (56.5388, 35.5228) construction
  line L5356 (56.5388, 35.5228) -> (56.629, 35.6577) construction
  line L5357 (56.629, 35.6577) -> (56.7185, 35.7933) construction
  line L5358 (56.7185, 35.7933) -> (56.8073, 35.9295) construction
  line L5359 (56.8073, 35.9295) -> (56.8955, 36.0665) construction
  line L5360 (56.8955, 36.0665) -> (56.9829, 36.2042) construction
  line L5361 (56.9829, 36.2042) -> (57.0697, 36.3425) construction
  line L5362 (57.0697, 36.3425) -> (57.1558, 36.4815) construction
  line L5363 (57.1558, 36.4815) -> (57.2413, 36.6211) construction
  line L5364 (57.2413, 36.6211) -> (57.3261, 36.7614) construction
  line L5365 (57.3261, 36.7614) -> (57.4102, 36.9023) construction
  line L5366 (57.4102, 36.9023) -> (57.4937, 37.0438) construction
  line L5367 (57.4937, 37.0438) -> (57.5765, 37.186) construction
  line L5368 (57.5765, 37.186) -> (57.6587, 37.3288) construction
  line L5369 (57.6587, 37.3288) -> (57.7403, 37.4721) construction
  line L5370 (57.7403, 37.4721) -> (57.8212, 37.6161) construction
  line L5371 (57.8212, 37.6161) -> (57.9014, 37.7607) construction
  line L5372 (57.9014, 37.7607) -> (57.981, 37.9058) construction
  line L5373 (57.981, 37.9058) -> (58.06, 38.0515) construction
  line L5374 (58.06, 38.0515) -> (58.1383, 38.1978) construction
  line L5375 (58.1383, 38.1978) -> (58.216, 38.3447) construction
  line L5376 (58.216, 38.3447) -> (58.2931, 38.4921) construction
  line L5377 (58.2931, 38.4921) -> (58.3695, 38.6401) construction
  line L5378 (58.3695, 38.6401) -> (58.4453, 38.7886) construction
  line L5379 (58.4453, 38.7886) -> (58.5205, 38.9377) construction
  line L5380 (58.5205, 38.9377) -> (58.595, 39.0873) construction
  line L5381 (58.595, 39.0873) -> (58.669, 39.2374) construction
  line L5382 (58.669, 39.2374) -> (58.7423, 39.3881) construction
  line L5383 (58.7423, 39.3881) -> (58.8149, 39.5393) construction
  line L5384 (58.8149, 39.5393) -> (58.887, 39.6909) construction
  line L5385 (58.887, 39.6909) -> (58.9584, 39.8431) construction
  line L5386 (58.9584, 39.8431) -> (59.0151, 39.9653) construction
  line L5387 (59.0151, 39.9653) -> (59.0573, 40.0572) construction
  line L5388 (59.0573, 40.0572) -> (59.0853, 40.1185) construction
  line L5389 (59.0853, 40.1185) -> (59.0993, 40.1492) construction
  arc A132 (-51.9354, -24.5301) -> (-50.3721, -27.5982) centre (0, 0) ccw
  line L5390 (23.5481, 54.5366) -> (24.1948, 56.0345)
  arc A133 (56.435, -10.6816) -> (56.9737, -7.2806) centre (0, 0) ccw
  line L5391 (39.2483, 44.5906) -> (40.3263, 45.8153)
  line L5392 (59.1442, -5.5428) -> (60.7685, -5.6951)
  line L5393 (44.5906, 39.2483) -> (45.8153, 40.3263)
  arc A134 (-50.3721, 27.5982) -> (-51.1066, 30.2798) centre (-52.1261, 28.5592) ccw
  arc A135 (-56.435, 10.6816) -> (-57.9623, 13.005) centre (-58.4001, 11.0535) ccw
  arc A136 (-13.005, 57.9623) -> (-10.6816, 56.435) centre (-11.0535, 58.4001) ccw
  spline S72 degree 5 poles (-45.8153, -40.3263) (-45.8385, -40.3467) (-45.8854, -40.3868) (-45.9573, -40.4451) (-46.056, -40.5192) (-46.1833, -40.6066) (-46.3135, -40.6904) (-46.4454, -40.772) (-46.5782, -40.8524) (-46.7117, -40.932) (-46.8458, -41.0107) (-46.9807, -41.0883) (-47.1168, -41.1642) (-47.2543, -41.2383) (-47.393, -41.3106) (-47.5329, -41.3813) (-47.6738, -41.4504) (-47.8156, -41.5184) (-47.9581, -41.5853) (-48.1012, -41.6512) (-48.245, -41.716) (-48.3895, -41.7798) (-48.5347, -41.8424) (-48.6807, -41.9039) (-48.8274, -41.9642) (-48.9749, -42.0234) (-49.123, -42.0815) (-49.2717, -42.1386) (-49.421, -42.1947) (-49.5709, -42.2499) (-49.7214, -42.3041) (-49.8724, -42.3574) (-50.024, -42.4097) (-50.1761, -42.461) (-50.3288, -42.5114) (-50.482, -42.5608) (-50.6358, -42.6094) (-50.79, -42.657) (-50.9447, -42.7037) (-51.0999, -42.7495) (-51.2556, -42.7945) (-51.4118, -42.8386) (-51.5684, -42.8818) (-51.7255, -42.9241) (-51.883, -42.9656) (-52.0409, -43.0063) (-52.1993, -43.0461) (-52.3581, -43.085) (-52.5173, -43.1231) (-52.6769, -43.1604) (-52.8369, -43.1969) (-52.9973, -43.2326) (-53.1581, -43.2674) (-53.3193, -43.3015) (-53.4809, -43.3347) (-53.6428, -43.3672) (-53.8051, -43.3988) (-53.9677, -43.4297) (-54.1307, -43.4597) (-54.294, -43.489) (-54.4577, -43.5175) (-54.6217, -43.5453) (-54.7861, -43.5723) (-54.9508, -43.5984) (-55.1158, -43.6239) (-55.2811, -43.6486) (-55.4467, -43.6725) (-55.6126, -43.6956) (-55.7789, -43.718) (-55.9454, -43.7397) (-56.1122, -43.7606) (-56.2459, -43.7767) (-56.3463, -43.7885) (-56.4133, -43.7962) (-56.4469, -43.8) knots 0 0 0 0 0 0 0.01428571 0.02857143 0.04285714 0.05714286 0.07142857 0.08571429 0.1 0.11428571 0.12857143 0.14285714 0.15714286 0.17142857 0.18571429 0.2 0.21428571 0.22857143 0.24285714 0.25714286 0.27142857 0.28571429 0.3 0.31428571 0.32857143 0.34285714 0.35714286 0.37142857 0.38571429 0.4 0.41428571 0.42857143 0.44285714 0.45714286 0.47142857 0.48571429 0.5 0.51428571 0.52857143 0.54285714 0.55714286 0.57142857 0.58571429 0.6 0.61428571 0.62857143 0.64285714 0.65714286 0.67142857 0.68571429 0.7 0.71428571 0.72857143 0.74285714 0.75714286 0.77142857 0.78571429 0.8 0.81428571 0.82857143 0.84285714 0.85714286 0.87142857 0.88571429 0.9 0.91428571 0.92857143 0.94285714 0.95714286 0.97142857 0.98571429 1 1 1 1 1 1
  line L5394 (-45.8153, -40.3263) -> (-45.8385, -40.3467) construction
  line L5395 (-45.8385, -40.3467) -> (-45.8854, -40.3868) construction
  line L5396 (-45.8854, -40.3868) -> (-45.9573, -40.4451) construction
  line L5397 (-45.9573, -40.4451) -> (-46.056, -40.5192) construction
  line L5398 (-46.056, -40.5192) -> (-46.1833, -40.6066) construction
  line L5399 (-46.1833, -40.6066) -> (-46.3135, -40.6904) construction
  line L5400 (-46.3135, -40.6904) -> (-46.4454, -40.772) construction
  line L5401 (-46.4454, -40.772) -> (-46.5782, -40.8524) construction
  line L5402 (-46.5782, -40.8524) -> (-46.7117, -40.932) construction
  line L5403 (-46.7117, -40.932) -> (-46.8458, -41.0107) construction
  line L5404 (-46.8458, -41.0107) -> (-46.9807, -41.0883) construction
  line L5405 (-46.9807, -41.0883) -> (-47.1168, -41.1642) construction
  line L5406 (-47.1168, -41.1642) -> (-47.2543, -41.2383) construction
  line L5407 (-47.2543, -41.2383) -> (-47.393, -41.3106) construction
  line L5408 (-47.393, -41.3106) -> (-47.5329, -41.3813) construction
  line L5409 (-47.5329, -41.3813) -> (-47.6738, -41.4504) construction
  line L5410 (-47.6738, -41.4504) -> (-47.8156, -41.5184) construction
  line L5411 (-47.8156, -41.5184) -> (-47.9581, -41.5853) construction
  line L5412 (-47.9581, -41.5853) -> (-48.1012, -41.6512) construction
  line L5413 (-48.1012, -41.6512) -> (-48.245, -41.716) construction
  line L5414 (-48.245, -41.716) -> (-48.3895, -41.7798) construction
  line L5415 (-48.3895, -41.7798) -> (-48.5347, -41.8424) construction
  line L5416 (-48.5347, -41.8424) -> (-48.6807, -41.9039) construction
  line L5417 (-48.6807, -41.9039) -> (-48.8274, -41.9642) construction
  line L5418 (-48.8274, -41.9642) -> (-48.9749, -42.0234) construction
  line L5419 (-48.9749, -42.0234) -> (-49.123, -42.0815) construction
  line L5420 (-49.123, -42.0815) -> (-49.2717, -42.1386) construction
  line L5421 (-49.2717, -42.1386) -> (-49.421, -42.1947) construction
  line L5422 (-49.421, -42.1947) -> (-49.5709, -42.2499) construction
  line L5423 (-49.5709, -42.2499) -> (-49.7214, -42.3041) construction
  line L5424 (-49.7214, -42.3041) -> (-49.8724, -42.3574) construction
  line L5425 (-49.8724, -42.3574) -> (-50.024, -42.4097) construction
  line L5426 (-50.024, -42.4097) -> (-50.1761, -42.461) construction
  line L5427 (-50.1761, -42.461) -> (-50.3288, -42.5114) construction
  line L5428 (-50.3288, -42.5114) -> (-50.482, -42.5608) construction
  line L5429 (-50.482, -42.5608) -> (-50.6358, -42.6094) construction
  line L5430 (-50.6358, -42.6094) -> (-50.79, -42.657) construction
  line L5431 (-50.79, -42.657) -> (-50.9447, -42.7037) construction
  line L5432 (-50.9447, -42.7037) -> (-51.0999, -42.7495) construction
  line L5433 (-51.0999, -42.7495) -> (-51.2556, -42.7945) construction
  line L5434 (-51.2556, -42.7945) -> (-51.4118, -42.8386) construction
  line L5435 (-51.4118, -42.8386) -> (-51.5684, -42.8818) construction
  line L5436 (-51.5684, -42.8818) -> (-51.7255, -42.9241) construction
  line L5437 (-51.7255, -42.9241) -> (-51.883, -42.9656) construction
  line L5438 (-51.883, -42.9656) -> (-52.0409, -43.0063) construction
  line L5439 (-52.0409, -43.0063) -> (-52.1993, -43.0461) construction
  line L5440 (-52.1993, -43.0461) -> (-52.3581, -43.085) construction
  line L5441 (-52.3581, -43.085) -> (-52.5173, -43.1231) construction
  line L5442 (-52.5173, -43.1231) -> (-52.6769, -43.1604) construction
  line L5443 (-52.6769, -43.1604) -> (-52.8369, -43.1969) construction
  line L5444 (-52.8369, -43.1969) -> (-52.9973, -43.2326) construction
  line L5445 (-52.9973, -43.2326) -> (-53.1581, -43.2674) construction
  line L5446 (-53.1581, -43.2674) -> (-53.3193, -43.3015) construction
  line L5447 (-53.3193, -43.3015) -> (-53.4809, -43.3347) construction
  line L5448 (-53.4809, -43.3347) -> (-53.6428, -43.3672) construction
  line L5449 (-53.6428, -43.3672) -> (-53.8051, -43.3988) construction
  line L5450 (-53.8051, -43.3988) -> (-53.9677, -43.4297) construction
  line L5451 (-53.9677, -43.4297) -> (-54.1307, -43.4597) construction
  line L5452 (-54.1307, -43.4597) -> (-54.294, -43.489) construction
  line L5453 (-54.294, -43.489) -> (-54.4577, -43.5175) construction
  line L5454 (-54.4577, -43.5175) -> (-54.6217, -43.5453) construction
  line L5455 (-54.6217, -43.5453) -> (-54.7861, -43.5723) construction
  line L5456 (-54.7861, -43.5723) -> (-54.9508, -43.5984) construction
  line L5457 (-54.9508, -43.5984) -> (-55.1158, -43.6239) construction
  line L5458 (-55.1158, -43.6239) -> (-55.2811, -43.6486) construction
  line L5459 (-55.2811, -43.6486) -> (-55.4467, -43.6725) construction
  line L5460 (-55.4467, -43.6725) -> (-55.6126, -43.6956) construction
  line L5461 (-55.6126, -43.6956) -> (-55.7789, -43.718) construction
  line L5462 (-55.7789, -43.718) -> (-55.9454, -43.7397) construction
  line L5463 (-55.9454, -43.7397) -> (-56.1122, -43.7606) construction
  line L5464 (-56.1122, -43.7606) -> (-56.2459, -43.7767) construction
  line L5465 (-56.2459, -43.7767) -> (-56.3463, -43.7885) construction
  line L5466 (-56.3463, -43.7885) -> (-56.4133, -43.7962) construction
  line L5467 (-56.4133, -43.7962) -> (-56.4469, -43.8) construction
  arc A137 (57.9623, 13.005) -> (56.435, 10.6816) centre (58.4001, 11.0535) ccw
  arc A138 (-23.5481, -54.5366) -> (-24.5301, -51.9354) centre (-25.3842, -53.7438) ccw